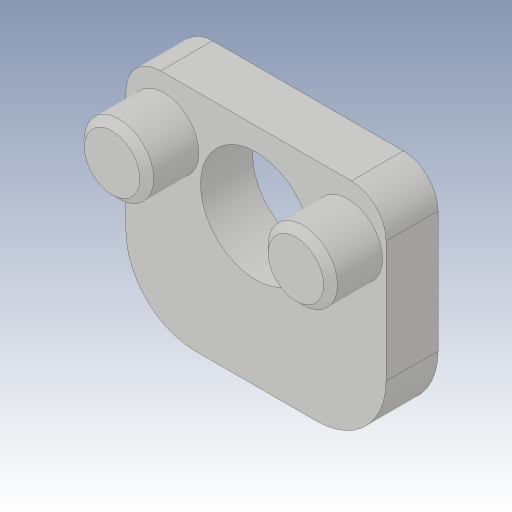
# Autodesk Inventor part: BT006_huenin20_23
Saved by Autodesk Inventor 2023.2 (Build 272271030, 271C)
## iProperties
Company: HTBLA Kaindorf
RuleStatus: InUse
Created: 2023-08-13
Part Number: BT006_huenin20_23
Project: Fiberprinter-Hotend
Material: Generisch
Description: Heatpadding_2
Document SubType Name: Modeling
Designer: huenin20
Density: 1 g/cm^3
Appearance: Vorgabe
Mass: 0.0670325 g
Surface Area: 1.47613 cm^2
Volume: 0.0670325 cm^3
AfterDocNew0: iProperties-Editor_aufrufen
Author: nicob
Keywords: 2023
Autodesk Inventor part; units mm, degrees
ref_plane "YZ Plane" through (0, 0, 0) normal (1, 0, 0) x (0, 1, 0)
ref_plane "XZ Plane" through (0, 0, 0) normal (0, 1, 0) x (-1, 0, 0)
ref_plane "XY Plane" through (0, 0, 0) normal (0, 0, 1) x (1, 0, 0)
sketch "Skizze3" plane through (0, 0, 0) normal (1, 0, 0) x (0, 1, 0)
  line L0 (0, 0) -> (-7.5, 0)
  line L1 (-7.5, 0) -> (-7.5, -4.5)
  line L2 (-5.5, -6.5) -> (-2, -6.5)
  line L3 (0, -4.5) -> (0, 0)
  arc A0 (-7.5, -4.5) -> (-5.5, -6.5) centre (-5.5, -4.5) ccw
  arc A1 (-2, -6.5) -> (0, -4.5) centre (-2, -4.5) ccw
  line L4 (-7.5, -1.5) -> (0, -1.5) construction
  circle A2 centre (-6.4, -1.5) radius 1
  circle A3 centre (-1.1, -1.5) radius 1
  circle A4 centre (-3.75, -2.25) radius 1.6
  point P0 (-7.5, -6.5)
  point P1 (0, -6.5)
  point P2 (0, -2.25)
  point P3 (-3.75, 0)
  dimension "d4" = 7.5
  dimension "d5" = 6.5
  dimension "d6" = 2
  dimension "d7" = 1.5
  dimension "d8" = 2
  dimension "d9" = 2
  dimension "d10" = 1.1
  dimension "d11" = 1.1
  dimension "d13" = 3.2
  dimension "d14" = 2.25
  constraints: 10 end point, 8 point on line, 5 centre point, 4 point on circle, 4 tangent, 2 horizontal, 2 midpoint, 2 parallel, 1 equal radius, 1 perpendicular, 1 vertical alignment
  measures "d4" distance of point (0, -6.5) point (-7.5, -6.5)
  measures "d5" distance of point (-7.5, -6.5) L0.end
  measures "d6" radius of A0
  measures "d7" distance between parallel lines of L0 L4
  measures "d8" diameter of A2
  measures "d9" diameter of A3
  measures "d10" horizontal distance of point (0, -2.25) A3.centre
  measures "d11" distance from line of L1 A2.centre
  measures "d13" diameter of A4
  measures "d14" distance from line of L0 A4.centre
extrude "Extrusion3" add sketch "Skizze3" against normal blind 1.5 contours L3 A1 L2 A0 L1 L0 | A2 | A3
extrude "Extrusion4" add sketch "Skizze3" along normal blind 1.5 contours A2 | A3
chamfer "Fase1" distance 0.2 angle 45 2 edges at (1.5, -2.1, -1.5) (1.5, -7.4, -1.5)
fillet "Rundung1" radius 1 2 edges at (-0.75, -7.5, 0) (-0.75, 0, 0)
equation "\"d11\" = d10"
